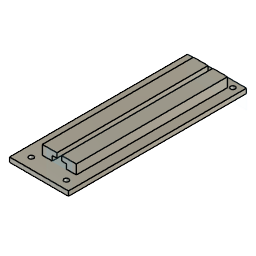
Rail System Demo 1 (Autodesk Fusion 360 design; units mm, degrees)
part number: 2025-10-30-15-29-35-854
Autodesk Fusion 360 part; units mm, degrees
sketch "Sketch1" plane through (0, 0, 0) normal (0, 0, 1) x (1, 0, 0)
  line L0 (-20, 30) -> (20.8523, 30)
  line L1 (20.8523, 30) -> (20.8523, -34.8194)
  line L2 (20.8523, -34.8194) -> (-20, -34.8194)
  line L3 (-20, -34.8194) -> (-20, 30)
  constraint horizontal L0
  constraint vertical L1
  constraint horizontal L2
  constraint vertical L3
sketch "Sketch2" plane through (0, 0, 0) normal (0, 0, 1) x (1, 0, 0)
  line L0 (-11.4066, 12.7433) -> (24.3229, 12.7433)
  line L1 (24.3229, 12.7433) -> (24.3229, -393.6567)
  line L2 (24.3229, -393.6567) -> (-11.4066, -393.6567)
  line L3 (-11.4066, -393.6567) -> (-11.4066, 12.7433)
  line L4 (-11.4066, 12.7433) -> (90.1934, 12.7433)
  line L5 (90.1934, 12.7433) -> (90.1934, -393.6567)
  line L6 (90.1934, -393.6567) -> (-11.4066, -393.6567)
  line L7 (-11.4066, -393.6567) -> (-11.4066, 12.7433)
  dimension "d3" = 406.4
  dimension "d4" = 101.6
  constraint horizontal L0
  constraint vertical L1
  constraint horizontal L2
  constraint vertical L3
  constraint horizontal L4
  constraint vertical L5
  constraint horizontal L6
  constraint vertical L7
  measures "d3" distance of L0.start L2.end
  measures "d4" distance of L0.start L4.end
extrude "Extrude2" add sketch "Sketch2" along normal blind 76.2 contours L1 L4 L5 L6
sketch "Sketch3" plane through (0, -393.6567, 0) normal (0, -1, 0) x (1, 0, 0)
  line L0 (24.3229, 0) -> (90.1934, 0)
  line L1 (90.1934, 0) -> (90.1934, 76.2)
  line L2 (90.1934, 76.2) -> (24.3229, 76.2)
  line L3 (24.3229, 76.2) -> (24.3229, 0)
sketch "Sketch4" plane through (0, -393.6567, 0) normal (0, -1, 0) x (1, 0, 0)
  line L0 (38.1, 63.5) -> (76.2, 63.5)
  line L1 (76.2, 63.5) -> (76.2, 50.8)
  line L2 (76.2, 50.8) -> (38.1, 50.8)
  line L3 (38.1, 50.8) -> (38.1, 63.5)
  constraint horizontal L0
  constraint vertical L1
  constraint horizontal L2
  constraint vertical L3
extrude "Extrude3" cut sketch "Sketch4" against normal blind 444.5
sketch "Sketch5" plane through (0, -393.6567, 0) normal (0, -1, 0) x (1, 0, 0)
  line L0 (50.8, 63.5) -> (63.5, 63.5)
  line L1 (63.5, 63.5) -> (63.5, 76.2)
  line L2 (63.5, 76.2) -> (50.8, 76.2)
  line L3 (50.8, 76.2) -> (50.8, 63.5)
  constraint horizontal L0
  constraint vertical L1
  constraint horizontal L2
  constraint vertical L3
extrude "Extrude4" cut sketch "Sketch5" against normal blind 419.1
sketch "Sketch6" plane through (0, 0, 76.2) normal (0, 0, 1) x (-1, 0, 0)
  line L0 (-50.8, 393.6567) -> (-50.8, -12.7433)
  line L1 (-50.8, -12.7433) -> (-24.3229, -12.7433)
  line L2 (-24.3229, -12.7433) -> (-24.3229, 393.6567)
  line L3 (-24.3229, 393.6567) -> (-50.8, 393.6567)
  line L4 (-6.8471, -24.8983) -> (-111.5412, -24.8983)
  line L5 (-111.5412, -24.8983) -> (-111.5412, 407.05)
  line L6 (-111.5412, 407.05) -> (-6.8471, 407.05)
  line L7 (-6.8471, 407.05) -> (-6.8471, -24.8983)
  circle A0 centre (-15.24, -17.78) radius 5.08
  circle A1 centre (-101.6, -17.78) radius 5.08
  circle A2 centre (-101.6, 398.78) radius 5.08
  circle A3 centre (-17.78, 398.78) radius 5.08
  point P0 (-12.7, 391.3931)
  dimension "d11" = 10.16
  dimension "d12" = 10.16
  constraint horizontal L4
  constraint vertical L5
  constraint horizontal L6
  constraint vertical L7
  measures "d11" diameter of A2
  measures "d12" diameter of A3
sketch "Sketch7" plane through (0, 0, 88.9) normal (0, 0, 1) x (-1, 0, 0)
sketch "Sketch8" plane through (0, 0, 0) normal (0, 0, -1) x (1, 0, 0)
  line L0 (24.3229, 393.6567) -> (24.3229, -12.7433)
  line L1 (24.3229, -12.7433) -> (90.1934, -12.7433)
  line L2 (90.1934, -12.7433) -> (90.1934, 393.6567)
  line L3 (90.1934, 393.6567) -> (24.3229, 393.6567)
  line L4 (129.5849, -37.1422) -> (-28.8884, -37.1422)
  line L5 (-28.8884, -37.1422) -> (-28.8884, 441.5791)
  line L6 (-28.8884, 441.5791) -> (129.5849, 441.5791)
  line L7 (129.5849, 441.5791) -> (129.5849, -37.1422)
  circle A0 centre (110.117, -19.8168) radius 6.35
  circle A1 centre (-6.6494, -18.0653) radius 6.35
  circle A2 centre (101.6, 419.1) radius 6.35
  circle A3 centre (0.9404, 412.8027) radius 6.35
  dimension "d15" = 12.7
  dimension "d16" = 12.7
  dimension "d17" = 12.7
  dimension "d18" = 12.7
  constraint horizontal L4
  constraint vertical L5
  constraint horizontal L6
  constraint vertical L7
  measures "d15" diameter of A0
  measures "d16" diameter of A1
  measures "d17" diameter of A2
  measures "d18" diameter of A3
extrude "Extrude6" add sketch "Sketch8" against normal blind 25.4
sketch "Sketch9" plane through (0, 0, 50.8) normal (0, 0, 1) x (-1, 0, 0)
  line L0 (-76.2, -12.7433) -> (-38.1, -12.7433)
  line L1 (-38.1, -12.7433) -> (-38.1, 393.6567)
  line L2 (-38.1, 393.6567) -> (-76.2, 393.6567)
  line L3 (-76.2, 393.6567) -> (-76.2, -12.7433)
extrude "Extrude7" add 1 faces at (14.3299, -123.04, 25.4) along direction (0, 0, 1) blind 25.4
sketch "Sketch10" plane through (0, -393.6567, 0) normal (0, -1, 0) x (1, 0, 0)
sketch "Sketch11" plane through (0, 37.1422, 0) normal (0, 1, 0) x (-1, 0, 0)
  line L0 (-129.5849, 0) -> (28.8884, 0)
  line L1 (28.8884, 0) -> (28.8884, 50.8)
  line L2 (28.8884, 50.8) -> (-129.5849, 50.8)
  line L3 (-129.5849, 50.8) -> (-129.5849, 0)
extrude "Extrude8" cut 1 faces at (35.4568, -126.9866, 0) along direction (0, 0, 1) blind 38.1
extrude "Extrude9" add 1 faces at (24.3229, -122.7234, 59.2667) along direction (-1, 0, 0) blind 12.7
extrude "Extrude10" add 1 faces at (90.1934, -122.7234, 59.2667) along direction (1, 0, 0) blind 12.7
